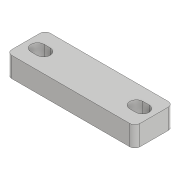
# Autodesk Inventor part: SoporteMancal
Saved by Autodesk Inventor 2022 (Build 260153000, 153)
## iProperties
Created: 2019-11-07
Part Number: SoporteMancal
Material: Genérico
Document SubType Name: Modeling
Designer: usuario_2
Density: 1 g/cm^3
Appearance: Valor por defecto
Author: usuario_2
Autodesk Inventor part; units mm, degrees
ref_plane "YZ Plane" through (0, 0, 0) normal (1, 0, 0) x (0, 1, 0)
ref_plane "XZ Plane" through (0, 0, 0) normal (0, 1, 0) x (-1, 0, 0)
ref_plane "XY Plane" through (0, 0, 0) normal (0, 0, 1) x (1, 0, 0)
sketch "Boceto1" plane through (0, 0, 0) normal (0, 0, 1) x (1, 0, 0)
  line L0 (-58.5, -19) -> (58.5, -19)
  line L1 (63.5, -14) -> (63.5, 14)
  line L2 (58.5, 19) -> (-58.5, 19)
  line L3 (-63.5, 14) -> (-63.5, -14)
  line L4 (-63.5, -19) -> (63.5, 19) construction
  line L5 (63.5, -19) -> (-63.5, 19) construction
  arc A0 (-58.5, 19) -> (-63.5, 14) centre (-58.5, 14) ccw
  arc A1 (-63.5, -14) -> (-58.5, -19) centre (-58.5, -14) ccw
  arc A2 (58.5, -19) -> (63.5, -14) centre (58.5, -14) ccw
  arc A3 (63.5, 14) -> (58.5, 19) centre (58.5, 14) ccw
  line L6 (-63.5, 0) -> (63.5, 0) construction
  line L7 (-58.5, 0) -> (-39.5, 0) construction
  line L8 (-52, -6.5) -> (-46, -6.5)
  line L9 (-46, 6.5) -> (-52, 6.5)
  arc A4 (-52, 6.5) -> (-52, -6.5) centre (-52, 0) ccw
  arc A5 (-46, -6.5) -> (-46, 6.5) centre (-46, 0) ccw
  line L10 (0, 19) -> (0, -19) construction
  line L11 (52, -6.5) -> (46, -6.5)
  line L12 (46, 6.5) -> (52, 6.5)
  arc A6 (52, -6.5) -> (52, 6.5) centre (52, 0) ccw
  arc A7 (46, 6.5) -> (46, -6.5) centre (46, 0) ccw
  point P0 (0, 0)
  point P1 (-49, 0)
  dimension "d0" = 38
  dimension "d1" = 127
  dimension "d2" = 5
  dimension "d3" = 5
  dimension "d4" = 19
  dimension "d6" = 13
  constraints: 28 end point, 18 point on circle, 12 point on line, 12 tangent, 8 centre point, 7 midpoint, 6 symmetric about line, 3 equal radius, 3 parallel, 1 horizontal, 1 perpendicular, 2 other
  measures "d0" distance of L5.start L4.end
  measures "d1" distance of L4.end L5.end
  measures "d2" radius of A0
  measures "d3" distance of L6.start L7.start
  measures "d4" distance of L7.end L7.start
  measures "d6" distance between parallel lines of L8 L9
extrude "Extrusión1" add sketch "Boceto1" along normal blind 20
